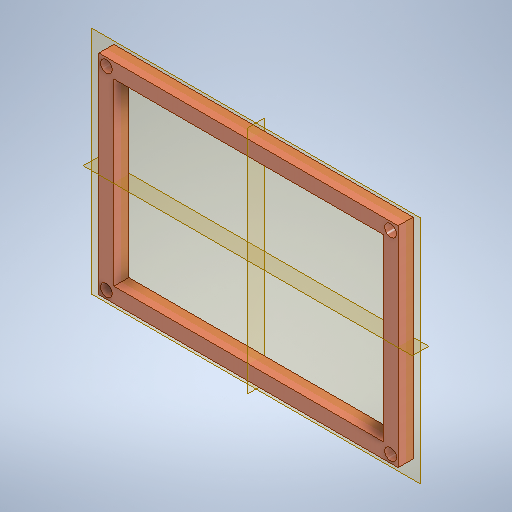
# Autodesk Inventor part: Mesa_001
Saved by Autodesk Inventor 2025.2 (Build 292293000, 293)
## iProperties
Created: 2025-04-07
Part Number: Mesa_001
Material: Madeira (Nogueira)
Document SubType Name: Modeling
Designer: Formação
Density: 0.55 g/cm^3
Appearance: Nogueira - Natural polido
Author: Formação
Autodesk Inventor part; units mm, degrees
sketch "Esboço1" plane through (0, 0, 0) normal (0, 0, 1) x (1, 0, 0)
  line L0 (-2500, 1750) -> (2500, 1750)
  line L1 (2500, 1750) -> (2500, -1750)
  line L2 (2500, -1750) -> (-2500, -1750)
  line L3 (-2500, -1750) -> (-2500, 1750)
  line L4 (-2500, 1750) -> (2500, -1750) construction
  line L5 (2500, 1750) -> (-2500, -1750) construction
  line L6 (-2250, 1500) -> (2250, 1500)
  line L7 (2250, 1500) -> (2250, -1500)
  line L8 (2250, -1500) -> (-2250, -1500)
  line L9 (-2250, -1500) -> (-2250, 1500)
  line L10 (-2250, 1500) -> (2250, -1500) construction
  line L11 (2250, 1500) -> (-2250, -1500) construction
  circle A0 centre (2375, 1620) radius 100
  circle A1 centre (2375, 1620) radius 75
  circle A2 centre (2375, -1620) radius 100
  circle A3 centre (2375, -1620) radius 75
  line L12 (2375, 1620) -> (2375, -1620) construction
  line L13 (2375, -1620) -> (-2375, -1620) construction
  line L14 (2375, 1620) -> (-2375, 1620) construction
  line L15 (-2375, 1620) -> (-2375, -1620) construction
  circle A4 centre (-2375, -1620) radius 100
  circle A5 centre (-2375, -1620) radius 75
  line L16 (-2375, 1620) -> (-2375, -1620) construction
  line L17 (-2375, -1620) -> (-5032.3735, -1620) construction
  circle A6 centre (-2375, 1620) radius 100
  circle A7 centre (-2375, 1620) radius 75
  line L18 (-2375, 4860) -> (-2375, 1620) construction
  line L19 (-2375, 1620) -> (-5788.4963, 1620) construction
  point P0 (0, 0)
  point P1 (0, 0)
  point P2 (0, 0)
  dimension "d0" = 5000
  dimension "d1" = 3500
  dimension "d2" = 250
  dimension "d3" = 250
  dimension "d6" = 200
  dimension "d8" = 125
  dimension "d9" = 120
  dimension "d10" = 25
  dimension "d11" = 200
  dimension "d12" = 25
  dimension "d16" = 125
  dimension "d18" = 120
  dimension "d19" = 200
  dimension "d20" = 25
  dimension "d21" = 200
  dimension "d22" = 25
  constraints: 40 end point, 13 coincident, 8 centre point, 6 parallel, 5 horizontal, 5 midpoint, 4 concentric, 3 horizontal alignment, 3 perpendicular, 1 vertical alignment
  measures "d0" distance of L0.end L0.start
  measures "d1" distance of L1.end L0.end
  measures "d2" distance between parallel lines of L0 L6
  measures "d3" distance between parallel lines of L1 L7
  measures "d6" diameter of A0
  measures "d8" distance from line of L1 A0.centre
  measures "d9" distance from line of L6 A0.centre
  measures "d10" radial gap between concentric circles of A0 A1
  measures "d11" diameter of A2
  measures "d12" radial gap between concentric circles of A2 A3
  measures "d16" distance from line of L3 L13.end
  measures "d18" vertical distance of L7.end A2.centre
  measures "d19" diameter of A4
  measures "d20" radial gap between concentric circles of A4 A5
  measures "d21" diameter of A6
  measures "d22" radial gap between concentric circles of A6 A7
extrude "Extrusão3" add sketch "Esboço1" along normal mid plane 250 contours L0 L1 L2 L3
